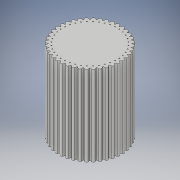
# Autodesk Inventor part: shaft
Saved by Autodesk Inventor 2019.3 (Build 233278000, 278)
## iProperties
Created: 2018-12-19
Part Number: shaft
Material: Generic
Document SubType Name: Modeling
Designer: Frienddo
Density: 1 g/cm^3
Appearance: Default
Author: Frienddo
Autodesk Inventor part; units mm, degrees
ref_plane "YZ Plane" through (0, 0, 0) normal (1, 0, 0) x (0, 1, 0)
ref_plane "XZ Plane" through (0, 0, 0) normal (0, 1, 0) x (-1, 0, 0)
ref_plane "XY Plane" through (0, 0, 0) normal (0, 0, 1) x (1, 0, 0)
sketch "Sketch1" plane through (0, 0, 0) normal (0, 1, 0) x (-1, 0, 0)
  line L0 (2.2915, -4.4974) -> (1.9316, -4.6633)
  line L1 (1.9316, -4.6633) -> (1.5598, -4.8005)
  line L2 (1.5598, -4.8005) -> (1.1783, -4.9081)
  line L3 (1.1783, -4.9081) -> (0.7896, -4.9854)
  line L4 (0.7896, -4.9854) -> (0.396, -5.032)
  line L5 (0.396, -5.032) -> (0, -5.0475)
  line L6 (0, -5.0475) -> (-0.396, -5.032)
  line L7 (-0.396, -5.032) -> (-0.7896, -4.9854)
  line L8 (-0.7896, -4.9854) -> (-1.1783, -4.9081)
  line L9 (-1.1783, -4.9081) -> (-1.5598, -4.8005)
  line L10 (-1.5598, -4.8005) -> (-1.9316, -4.6633)
  line L11 (-1.9316, -4.6633) -> (-2.2915, -4.4974)
  line L12 (-2.2915, -4.4974) -> (-2.6373, -4.3037)
  line L13 (-2.6373, -4.3037) -> (-2.9669, -4.0835)
  line L14 (-2.9669, -4.0835) -> (-3.2781, -3.8382)
  line L15 (-3.2781, -3.8382) -> (-3.5692, -3.5692)
  line L16 (-3.5692, -3.5692) -> (-3.8382, -3.2781)
  line L17 (-3.8382, -3.2781) -> (-4.0835, -2.9669)
  line L18 (-4.0835, -2.9669) -> (-4.3037, -2.6373)
  line L19 (-4.3037, -2.6373) -> (-4.4974, -2.2915)
  line L20 (-4.4974, -2.2915) -> (-4.6633, -1.9316)
  line L21 (-4.6633, -1.9316) -> (-4.8005, -1.5598)
  line L22 (-4.8005, -1.5598) -> (-4.9081, -1.1783)
  line L23 (-4.9081, -1.1783) -> (-4.9854, -0.7896)
  line L24 (-4.9854, -0.7896) -> (-5.032, -0.396)
  line L25 (-5.032, -0.396) -> (-5.0475, 0)
  line L26 (-5.0475, 0) -> (-5.032, 0.396)
  line L27 (-5.032, 0.396) -> (-4.9854, 0.7896)
  line L28 (-4.9854, 0.7896) -> (-4.9081, 1.1783)
  line L29 (-4.9081, 1.1783) -> (-4.8005, 1.5598)
  line L30 (-4.8005, 1.5598) -> (-4.6633, 1.9316)
  line L31 (-4.6633, 1.9316) -> (-4.4974, 2.2915)
  line L32 (-4.4974, 2.2915) -> (-4.3037, 2.6373)
  line L33 (-4.3037, 2.6373) -> (-4.0835, 2.9669)
  line L34 (-4.0835, 2.9669) -> (-3.8382, 3.2781)
  line L35 (-3.8382, 3.2781) -> (-3.5692, 3.5692)
  line L36 (-3.5692, 3.5692) -> (-3.2781, 3.8382)
  line L37 (-3.2781, 3.8382) -> (-2.9669, 4.0835)
  line L38 (-2.9669, 4.0835) -> (-2.6373, 4.3037)
  line L39 (-2.6373, 4.3037) -> (-2.2915, 4.4974)
  line L40 (-2.2915, 4.4974) -> (-1.9316, 4.6633)
  line L41 (-1.9316, 4.6633) -> (-1.5598, 4.8005)
  line L42 (-1.5598, 4.8005) -> (-1.1783, 4.9081)
  line L43 (-1.1783, 4.9081) -> (-0.7896, 4.9854)
  line L44 (-0.7896, 4.9854) -> (-0.396, 5.032)
  line L45 (-0.396, 5.032) -> (0, 5.0475)
  line L46 (0, 5.0475) -> (0.396, 5.032)
  line L47 (0.396, 5.032) -> (0.7896, 4.9854)
  line L48 (0.7896, 4.9854) -> (1.1783, 4.9081)
  line L49 (1.1783, 4.9081) -> (1.5598, 4.8005)
  line L50 (1.5598, 4.8005) -> (1.9316, 4.6633)
  line L51 (1.9316, 4.6633) -> (2.2915, 4.4974)
  line L52 (2.2915, 4.4974) -> (2.6373, 4.3037)
  line L53 (2.6373, 4.3037) -> (2.9669, 4.0835)
  line L54 (2.9669, 4.0835) -> (3.2781, 3.8382)
  line L55 (3.2781, 3.8382) -> (3.5692, 3.5692)
  line L56 (3.5692, 3.5692) -> (3.8382, 3.2781)
  line L57 (3.8382, 3.2781) -> (4.0835, 2.9669)
  line L58 (4.0835, 2.9669) -> (4.3037, 2.6373)
  line L59 (4.3037, 2.6373) -> (4.4974, 2.2915)
  line L60 (4.4974, 2.2915) -> (4.6633, 1.9316)
  line L61 (4.6633, 1.9316) -> (4.8005, 1.5598)
  line L62 (4.8005, 1.5598) -> (4.9081, 1.1783)
  line L63 (4.9081, 1.1783) -> (4.9854, 0.7896)
  line L64 (4.9854, 0.7896) -> (5.032, 0.396)
  line L65 (5.032, 0.396) -> (5.0475, 0)
  line L66 (5.0475, 0) -> (5.032, -0.396)
  line L67 (5.032, -0.396) -> (4.9854, -0.7896)
  line L68 (4.9854, -0.7896) -> (4.9081, -1.1783)
  line L69 (4.9081, -1.1783) -> (4.8005, -1.5598)
  line L70 (4.8005, -1.5598) -> (4.6633, -1.9316)
  line L71 (4.6633, -1.9316) -> (4.4974, -2.2915)
  line L72 (4.4974, -2.2915) -> (4.3037, -2.6373)
  line L73 (4.3037, -2.6373) -> (4.0835, -2.9669)
  line L74 (4.0835, -2.9669) -> (3.8382, -3.2781)
  line L75 (3.8382, -3.2781) -> (3.5692, -3.5692)
  line L76 (3.5692, -3.5692) -> (3.2781, -3.8382)
  line L77 (3.2781, -3.8382) -> (2.9669, -4.0835)
  line L78 (2.9669, -4.0835) -> (2.6373, -4.3037)
  line L79 (2.6373, -4.3037) -> (2.2915, -4.4974)
  line L80 (0, 0) -> (0, -5.0475) construction
  circle A0 centre (0, -5.0475) radius 0.25
  circle A1 centre (-0.7896, -4.9854) radius 0.25
  circle A2 centre (-0.4486, -5.7003) radius 0.25
  line L81 (0, -5.0475) -> (-0.4486, -5.7003) construction
  line L82 (-0.4486, -5.7003) -> (-0.7896, -4.9854) construction
  line L83 (-0.4486, -5.7003) -> (0, 0) construction
  line L84 (0.206, -5.1891) -> (-0.2426, -5.8419)
  line L85 (-0.206, -4.9059) -> (-0.6547, -5.5587)
  line L86 (-0.223, -5.5927) -> (-0.564, -4.8778)
  line L87 (-0.6743, -5.8079) -> (-1.0153, -5.093)
  line L88 (0, 0) -> (0.4486, -5.7003) construction
  circle A3 centre (0.4486, -5.7003) radius 0.25
  line L89 (-0.206, -5.1891) -> (0, -5.4889)
  line L90 (0.6547, -5.5587) -> (0.206, -4.9059)
  line L91 (0, -5.0475) -> (0.4486, -5.7003) construction
  line L92 (0, -5.4889) -> (0.2426, -5.8419)
  circle A4 centre (0, 0) radius 3.4236 construction
  circle A5 centre (0, 0) radius 3.4236 construction
  circle A6 centre (1.3348, -5.5599) radius 0.25
  line L93 (0.8587, -5.4213) -> (1.1535, -5.732)
  line L94 (1.5162, -5.3878) -> (0.971, -4.8133)
  line L95 (1.0153, -5.093) -> (0.6743, -5.8079)
  line L96 (0.6083, -5.1575) -> (0.8587, -5.4213)
  circle A7 centre (0.7896, -4.9854) radius 0.25
  line L97 (0.564, -4.8778) -> (0.223, -5.5927)
  circle A8 centre (0.4486, -5.7003) radius 0.25
  circle A9 centre (0, 0) radius 3.4236 construction
  circle A10 centre (2.1882, -5.2827) radius 0.25
  line L98 (1.6962, -5.2203) -> (2.036, -5.481)
  line L99 (2.3403, -5.0843) -> (1.712, -4.6022)
  line L100 (1.7995, -4.8715) -> (1.5745, -5.6309)
  line L101 (1.4076, -4.9988) -> (1.6962, -5.2203)
  circle A11 centre (1.5598, -4.8005) radius 0.25
  line L102 (1.3201, -4.7295) -> (1.0951, -5.4889)
  circle A12 centre (1.3348, -5.5599) radius 0.25
  circle A13 centre (0, 0) radius 3.4236 construction
  circle A14 centre (2.9876, -4.8753) radius 0.25
  line L103 (2.4919, -4.8907) -> (2.8683, -5.095)
  line L104 (3.1069, -4.6556) -> (2.4108, -4.2777)
  line L105 (2.5394, -4.53) -> (2.436, -5.3153)
  line L106 (2.1722, -4.7171) -> (2.4919, -4.8907)
  circle A15 centre (2.2915, -4.4974) radius 0.25
  line L107 (2.0437, -4.4648) -> (1.9403, -5.25)
  circle A16 centre (2.1882, -5.2827) radius 0.25
  circle A17 centre (0, 0) radius 3.4236 construction
  circle A18 centre (3.7135, -4.3479) radius 0.25
  line L108 (3.2263, -4.4406) -> (3.63, -4.5836)
  line L109 (3.7969, -4.1123) -> (3.0503, -3.8479)
  line L110 (3.2168, -4.077) -> (3.2375, -4.8688)
  line L111 (2.8834, -4.3192) -> (3.2263, -4.4406)
  circle A19 centre (2.9669, -4.0835) radius 0.25
  line L112 (2.717, -4.0901) -> (2.7377, -4.8819)
  circle A20 centre (2.9876, -4.8753) radius 0.25
  circle A21 centre (0, 0) radius 3.4236 construction
  circle A22 centre (4.3479, -3.7135) radius 0.25
  line L113 (3.8813, -3.8813) -> (4.3024, -3.9593)
  line L114 (4.3935, -3.4677) -> (3.6147, -3.3233)
  line L115 (3.815, -3.5236) -> (3.9593, -4.3024)
  line L116 (3.5236, -3.815) -> (3.8813, -3.8813)
  circle A23 centre (3.5692, -3.5692) radius 0.25
  line L117 (3.3233, -3.6147) -> (3.4677, -4.3935)
  circle A24 centre (3.7135, -4.3479) radius 0.25
  circle A25 centre (0, 0) radius 3.4236 construction
  circle A26 centre (4.8753, -2.9876) radius 0.25
  line L118 (4.4406, -3.2263) -> (4.8688, -3.2375)
  line L119 (4.8819, -2.7377) -> (4.0901, -2.717)
  line L120 (4.3192, -2.8834) -> (4.5836, -3.63)
  line L121 (4.077, -3.2168) -> (4.4406, -3.2263)
  circle A27 centre (4.0835, -2.9669) radius 0.25
  line L122 (3.8479, -3.0503) -> (4.1123, -3.7969)
  circle A28 centre (4.3479, -3.7135) radius 0.25
  circle A29 centre (0, 0) radius 3.4236 construction
  circle A30 centre (5.2827, -2.1882) radius 0.25
  line L123 (4.8907, -2.4919) -> (5.3153, -2.436)
  line L124 (5.25, -1.9403) -> (4.4648, -2.0437)
  line L125 (4.7171, -2.1722) -> (5.095, -2.8683)
  line L126 (4.53, -2.5394) -> (4.8907, -2.4919)
  circle A31 centre (4.4974, -2.2915) radius 0.25
  line L127 (4.2777, -2.4108) -> (4.6556, -3.1069)
  circle A32 centre (4.8753, -2.9876) radius 0.25
  circle A33 centre (0, 0) radius 3.4236 construction
  circle A34 centre (5.5599, -1.3348) radius 0.25
  line L128 (5.2203, -1.6962) -> (5.6309, -1.5745)
  line L129 (5.4889, -1.0951) -> (4.7295, -1.3201)
  line L130 (4.9988, -1.4076) -> (5.481, -2.036)
  line L131 (4.8715, -1.7995) -> (5.2203, -1.6962)
  circle A35 centre (4.8005, -1.5598) radius 0.25
  line L132 (4.6022, -1.712) -> (5.0843, -2.3403)
  circle A36 centre (5.2827, -2.1882) radius 0.25
  circle A37 centre (0, 0) radius 3.4236 construction
  circle A38 centre (5.7003, -0.4486) radius 0.25
  line L133 (5.4213, -0.8587) -> (5.8079, -0.6743)
  line L134 (5.5927, -0.223) -> (4.8778, -0.564)
  line L135 (5.1575, -0.6083) -> (5.732, -1.1535)
  line L136 (5.093, -1.0153) -> (5.4213, -0.8587)
  circle A39 centre (4.9854, -0.7896) radius 0.25
  line L137 (4.8133, -0.971) -> (5.3878, -1.5162)
  circle A40 centre (5.5599, -1.3348) radius 0.25
  circle A41 centre (0, 0) radius 3.4236 construction
  circle A42 centre (5.7003, 0.4486) radius 0.25
  line L138 (5.4889, 0) -> (5.8419, 0.2426)
  line L139 (5.5587, 0.6547) -> (4.9059, 0.206)
  line L140 (5.1891, 0.206) -> (5.8419, -0.2426)
  line L141 (5.1891, -0.206) -> (5.4889, 0)
  circle A43 centre (5.0475, 0) radius 0.25
  line L142 (4.9059, -0.206) -> (5.5587, -0.6547)
  circle A44 centre (5.7003, -0.4486) radius 0.25
  circle A45 centre (0, 0) radius 3.4236 construction
  circle A46 centre (5.5599, 1.3348) radius 0.25
  line L143 (5.4213, 0.8587) -> (5.732, 1.1535)
  line L144 (5.3878, 1.5162) -> (4.8133, 0.971)
  line L145 (5.093, 1.0153) -> (5.8079, 0.6743)
  line L146 (5.1575, 0.6083) -> (5.4213, 0.8587)
  circle A47 centre (4.9854, 0.7896) radius 0.25
  line L147 (4.8778, 0.564) -> (5.5927, 0.223)
  circle A48 centre (5.7003, 0.4486) radius 0.25
  circle A49 centre (0, 0) radius 3.4236 construction
  circle A50 centre (5.2827, 2.1882) radius 0.25
  line L148 (5.2203, 1.6962) -> (5.481, 2.036)
  line L149 (5.0843, 2.3403) -> (4.6022, 1.712)
  line L150 (4.8715, 1.7995) -> (5.6309, 1.5745)
  line L151 (4.9988, 1.4076) -> (5.2203, 1.6962)
  circle A51 centre (4.8005, 1.5598) radius 0.25
  line L152 (4.7295, 1.3201) -> (5.4889, 1.0951)
  circle A52 centre (5.5599, 1.3348) radius 0.25
  circle A53 centre (0, 0) radius 3.4236 construction
  circle A54 centre (4.8753, 2.9876) radius 0.25
  line L153 (4.8907, 2.4919) -> (5.095, 2.8683)
  line L154 (4.6556, 3.1069) -> (4.2777, 2.4108)
  line L155 (4.53, 2.5394) -> (5.3153, 2.436)
  line L156 (4.7171, 2.1722) -> (4.8907, 2.4919)
  circle A55 centre (4.4974, 2.2915) radius 0.25
  line L157 (4.4648, 2.0437) -> (5.25, 1.9403)
  circle A56 centre (5.2827, 2.1882) radius 0.25
  circle A57 centre (0, 0) radius 3.4236 construction
  circle A58 centre (4.3479, 3.7135) radius 0.25
  line L158 (4.4406, 3.2263) -> (4.5836, 3.63)
  line L159 (4.1123, 3.7969) -> (3.8479, 3.0503)
  line L160 (4.077, 3.2168) -> (4.8688, 3.2375)
  line L161 (4.3192, 2.8834) -> (4.4406, 3.2263)
  circle A59 centre (4.0835, 2.9669) radius 0.25
  line L162 (4.0901, 2.717) -> (4.8819, 2.7377)
  circle A60 centre (4.8753, 2.9876) radius 0.25
  circle A61 centre (0, 0) radius 3.4236 construction
  circle A62 centre (3.7135, 4.3479) radius 0.25
  line L163 (3.8813, 3.8813) -> (3.9593, 4.3024)
  line L164 (3.4677, 4.3935) -> (3.3233, 3.6147)
  line L165 (3.5236, 3.815) -> (4.3024, 3.9593)
  line L166 (3.815, 3.5236) -> (3.8813, 3.8813)
  circle A63 centre (3.5692, 3.5692) radius 0.25
  line L167 (3.6147, 3.3233) -> (4.3935, 3.4677)
  circle A64 centre (4.3479, 3.7135) radius 0.25
  circle A65 centre (0, 0) radius 3.4236 construction
  circle A66 centre (2.9876, 4.8753) radius 0.25
  line L168 (3.2263, 4.4406) -> (3.2375, 4.8688)
  line L169 (2.7377, 4.8819) -> (2.717, 4.0901)
  line L170 (2.8834, 4.3192) -> (3.63, 4.5836)
  line L171 (3.2168, 4.077) -> (3.2263, 4.4406)
  circle A67 centre (2.9669, 4.0835) radius 0.25
  line L172 (3.0503, 3.8479) -> (3.7969, 4.1123)
  circle A68 centre (3.7135, 4.3479) radius 0.25
  circle A69 centre (0, 0) radius 3.4236 construction
  circle A70 centre (2.1882, 5.2827) radius 0.25
  line L173 (2.4919, 4.8907) -> (2.436, 5.3153)
  line L174 (1.9403, 5.25) -> (2.0437, 4.4648)
  line L175 (2.1722, 4.7171) -> (2.8683, 5.095)
  line L176 (2.5394, 4.53) -> (2.4919, 4.8907)
  circle A71 centre (2.2915, 4.4974) radius 0.25
  line L177 (2.4108, 4.2777) -> (3.1069, 4.6556)
  circle A72 centre (2.9876, 4.8753) radius 0.25
  circle A73 centre (0, 0) radius 3.4236 construction
  circle A74 centre (1.3348, 5.5599) radius 0.25
  line L178 (1.6962, 5.2203) -> (1.5745, 5.6309)
  line L179 (1.0951, 5.4889) -> (1.3201, 4.7295)
  line L180 (1.4076, 4.9988) -> (2.036, 5.481)
  line L181 (1.7995, 4.8715) -> (1.6962, 5.2203)
  circle A75 centre (1.5598, 4.8005) radius 0.25
  line L182 (1.712, 4.6022) -> (2.3403, 5.0843)
  circle A76 centre (2.1882, 5.2827) radius 0.25
  circle A77 centre (0, 0) radius 3.4236 construction
  circle A78 centre (0.4486, 5.7003) radius 0.25
  line L183 (0.8587, 5.4213) -> (0.6743, 5.8079)
  line L184 (0.223, 5.5927) -> (0.564, 4.8778)
  line L185 (0.6083, 5.1575) -> (1.1535, 5.732)
  line L186 (1.0153, 5.093) -> (0.8587, 5.4213)
  circle A79 centre (0.7896, 4.9854) radius 0.25
  line L187 (0.971, 4.8133) -> (1.5162, 5.3878)
  circle A80 centre (1.3348, 5.5599) radius 0.25
  circle A81 centre (0, 0) radius 3.4236 construction
  circle A82 centre (-0.4486, 5.7003) radius 0.25
  line L188 (0, 5.4889) -> (-0.2426, 5.8419)
  line L189 (-0.6547, 5.5587) -> (-0.206, 4.9059)
  line L190 (-0.206, 5.1891) -> (0.2426, 5.8419)
  line L191 (0.206, 5.1891) -> (0, 5.4889)
  circle A83 centre (0, 5.0475) radius 0.25
  line L192 (0.206, 4.9059) -> (0.6547, 5.5587)
  circle A84 centre (0.4486, 5.7003) radius 0.25
  circle A85 centre (0, 0) radius 3.4236 construction
  circle A86 centre (-1.3348, 5.5599) radius 0.25
  line L193 (-0.8587, 5.4213) -> (-1.1535, 5.732)
  line L194 (-1.5162, 5.3878) -> (-0.971, 4.8133)
  line L195 (-1.0153, 5.093) -> (-0.6743, 5.8079)
  line L196 (-0.6083, 5.1575) -> (-0.8587, 5.4213)
  circle A87 centre (-0.7896, 4.9854) radius 0.25
  line L197 (-0.564, 4.8778) -> (-0.223, 5.5927)
  circle A88 centre (-0.4486, 5.7003) radius 0.25
  circle A89 centre (0, 0) radius 3.4236 construction
  circle A90 centre (-2.1882, 5.2827) radius 0.25
  line L198 (-1.6962, 5.2203) -> (-2.036, 5.481)
  line L199 (-2.3403, 5.0843) -> (-1.712, 4.6022)
  line L200 (-1.7995, 4.8715) -> (-1.5745, 5.6309)
  line L201 (-1.4076, 4.9988) -> (-1.6962, 5.2203)
  circle A91 centre (-1.5598, 4.8005) radius 0.25
  line L202 (-1.3201, 4.7295) -> (-1.0951, 5.4889)
  circle A92 centre (-1.3348, 5.5599) radius 0.25
  circle A93 centre (0, 0) radius 3.4236 construction
  circle A94 centre (-2.9876, 4.8753) radius 0.25
  line L203 (-2.4919, 4.8907) -> (-2.8683, 5.095)
  line L204 (-3.1069, 4.6556) -> (-2.4108, 4.2777)
  line L205 (-2.5394, 4.53) -> (-2.436, 5.3153)
  line L206 (-2.1722, 4.7171) -> (-2.4919, 4.8907)
  circle A95 centre (-2.2915, 4.4974) radius 0.25
  line L207 (-2.0437, 4.4648) -> (-1.9403, 5.25)
  circle A96 centre (-2.1882, 5.2827) radius 0.25
  circle A97 centre (0, 0) radius 3.4236 construction
  circle A98 centre (-3.7135, 4.3479) radius 0.25
  line L208 (-3.2263, 4.4406) -> (-3.63, 4.5836)
  line L209 (-3.7969, 4.1123) -> (-3.0503, 3.8479)
  line L210 (-3.2168, 4.077) -> (-3.2375, 4.8688)
  line L211 (-2.8834, 4.3192) -> (-3.2263, 4.4406)
  circle A99 centre (-2.9669, 4.0835) radius 0.25
  line L212 (-2.717, 4.0901) -> (-2.7377, 4.8819)
  circle A100 centre (-2.9876, 4.8753) radius 0.25
  circle A101 centre (0, 0) radius 3.4236 construction
  circle A102 centre (-4.3479, 3.7135) radius 0.25
  line L213 (-3.8813, 3.8813) -> (-4.3024, 3.9593)
  line L214 (-4.3935, 3.4677) -> (-3.6147, 3.3233)
  line L215 (-3.815, 3.5236) -> (-3.9593, 4.3024)
  line L216 (-3.5236, 3.815) -> (-3.8813, 3.8813)
  circle A103 centre (-3.5692, 3.5692) radius 0.25
  line L217 (-3.3233, 3.6147) -> (-3.4677, 4.3935)
  circle A104 centre (-3.7135, 4.3479) radius 0.25
  circle A105 centre (0, 0) radius 3.4236 construction
  circle A106 centre (-4.8753, 2.9876) radius 0.25
  line L218 (-4.4406, 3.2263) -> (-4.8688, 3.2375)
  line L219 (-4.8819, 2.7377) -> (-4.0901, 2.717)
  line L220 (-4.3192, 2.8834) -> (-4.5836, 3.63)
  line L221 (-4.077, 3.2168) -> (-4.4406, 3.2263)
  circle A107 centre (-4.0835, 2.9669) radius 0.25
  line L222 (-3.8479, 3.0503) -> (-4.1123, 3.7969)
  circle A108 centre (-4.3479, 3.7135) radius 0.25
  circle A109 centre (0, 0) radius 3.4236 construction
  circle A110 centre (-5.2827, 2.1882) radius 0.25
  line L223 (-4.8907, 2.4919) -> (-5.3153, 2.436)
  line L224 (-5.25, 1.9403) -> (-4.4648, 2.0437)
  line L225 (-4.7171, 2.1722) -> (-5.095, 2.8683)
  line L226 (-4.53, 2.5394) -> (-4.8907, 2.4919)
  circle A111 centre (-4.4974, 2.2915) radius 0.25
  line L227 (-4.2777, 2.4108) -> (-4.6556, 3.1069)
  circle A112 centre (-4.8753, 2.9876) radius 0.25
  circle A113 centre (0, 0) radius 3.4236 construction
  circle A114 centre (-5.5599, 1.3348) radius 0.25
  line L228 (-5.2203, 1.6962) -> (-5.6309, 1.5745)
  line L229 (-5.4889, 1.0951) -> (-4.7295, 1.3201)
  line L230 (-4.9988, 1.4076) -> (-5.481, 2.036)
  line L231 (-4.8715, 1.7995) -> (-5.2203, 1.6962)
  circle A115 centre (-4.8005, 1.5598) radius 0.25
  line L232 (-4.6022, 1.712) -> (-5.0843, 2.3403)
  circle A116 centre (-5.2827, 2.1882) radius 0.25
  circle A117 centre (0, 0) radius 3.4236 construction
  circle A118 centre (-5.7003, 0.4486) radius 0.25
  line L233 (-5.4213, 0.8587) -> (-5.8079, 0.6743)
  line L234 (-5.5927, 0.223) -> (-4.8778, 0.564)
  line L235 (-5.1575, 0.6083) -> (-5.732, 1.1535)
  line L236 (-5.093, 1.0153) -> (-5.4213, 0.8587)
  circle A119 centre (-4.9854, 0.7896) radius 0.25
  line L237 (-4.8133, 0.971) -> (-5.3878, 1.5162)
  circle A120 centre (-5.5599, 1.3348) radius 0.25
  circle A121 centre (0, 0) radius 3.4236 construction
  circle A122 centre (-5.7003, -0.4486) radius 0.25
  line L238 (-5.4889, 0) -> (-5.8419, -0.2426)
  line L239 (-5.5587, -0.6547) -> (-4.9059, -0.206)
  line L240 (-5.1891, -0.206) -> (-5.8419, 0.2426)
  line L241 (-5.1891, 0.206) -> (-5.4889, 0)
  circle A123 centre (-5.0475, 0) radius 0.25
  line L242 (-4.9059, 0.206) -> (-5.5587, 0.6547)
  circle A124 centre (-5.7003, 0.4486) radius 0.25
  circle A125 centre (0, 0) radius 3.4236 construction
  circle A126 centre (-5.5599, -1.3348) radius 0.25
  line L243 (-5.4213, -0.8587) -> (-5.732, -1.1535)
  line L244 (-5.3878, -1.5162) -> (-4.8133, -0.971)
  line L245 (-5.093, -1.0153) -> (-5.8079, -0.6743)
  line L246 (-5.1575, -0.6083) -> (-5.4213, -0.8587)
  circle A127 centre (-4.9854, -0.7896) radius 0.25
  line L247 (-4.8778, -0.564) -> (-5.5927, -0.223)
  circle A128 centre (-5.7003, -0.4486) radius 0.25
  circle A129 centre (0, 0) radius 3.4236 construction
  circle A130 centre (-5.2827, -2.1882) radius 0.25
  line L248 (-5.2203, -1.6962) -> (-5.481, -2.036)
  line L249 (-5.0843, -2.3403) -> (-4.6022, -1.712)
  line L250 (-4.8715, -1.7995) -> (-5.6309, -1.5745)
  line L251 (-4.9988, -1.4076) -> (-5.2203, -1.6962)
  circle A131 centre (-4.8005, -1.5598) radius 0.25
  line L252 (-4.7295, -1.3201) -> (-5.4889, -1.0951)
  circle A132 centre (-5.5599, -1.3348) radius 0.25
  circle A133 centre (0, 0) radius 3.4236 construction
  circle A134 centre (-4.8753, -2.9876) radius 0.25
  line L253 (-4.8907, -2.4919) -> (-5.095, -2.8683)
  line L254 (-4.6556, -3.1069) -> (-4.2777, -2.4108)
  line L255 (-4.53, -2.5394) -> (-5.3153, -2.436)
  line L256 (-4.7171, -2.1722) -> (-4.8907, -2.4919)
  circle A135 centre (-4.4974, -2.2915) radius 0.25
  line L257 (-4.4648, -2.0437) -> (-5.25, -1.9403)
  circle A136 centre (-5.2827, -2.1882) radius 0.25
  circle A137 centre (0, 0) radius 3.4236 construction
  circle A138 centre (-4.3479, -3.7135) radius 0.25
  line L258 (-4.4406, -3.2263) -> (-4.5836, -3.63)
  line L259 (-4.1123, -3.7969) -> (-3.8479, -3.0503)
  line L260 (-4.077, -3.2168) -> (-4.8688, -3.2375)
  line L261 (-4.3192, -2.8834) -> (-4.4406, -3.2263)
  circle A139 centre (-4.0835, -2.9669) radius 0.25
  line L262 (-4.0901, -2.717) -> (-4.8819, -2.7377)
  circle A140 centre (-4.8753, -2.9876) radius 0.25
  circle A141 centre (0, 0) radius 3.4236 construction
  circle A142 centre (-3.7135, -4.3479) radius 0.25
  line L263 (-3.8813, -3.8813) -> (-3.9593, -4.3024)
  line L264 (-3.4677, -4.3935) -> (-3.3233, -3.6147)
  line L265 (-3.5236, -3.815) -> (-4.3024, -3.9593)
  line L266 (-3.815, -3.5236) -> (-3.8813, -3.8813)
  circle A143 centre (-3.5692, -3.5692) radius 0.25
  line L267 (-3.6147, -3.3233) -> (-4.3935, -3.4677)
  circle A144 centre (-4.3479, -3.7135) radius 0.25
  circle A145 centre (0, 0) radius 3.4236 construction
  circle A146 centre (-2.9876, -4.8753) radius 0.25
  line L268 (-3.2263, -4.4406) -> (-3.2375, -4.8688)
  line L269 (-2.7377, -4.8819) -> (-2.717, -4.0901)
  line L270 (-2.8834, -4.3192) -> (-3.63, -4.5836)
  line L271 (-3.2168, -4.077) -> (-3.2263, -4.4406)
  circle A147 centre (-2.9669, -4.0835) radius 0.25
  line L272 (-3.0503, -3.8479) -> (-3.7969, -4.1123)
  circle A148 centre (-3.7135, -4.3479) radius 0.25
  circle A149 centre (0, 0) radius 3.4236 construction
  circle A150 centre (-2.1882, -5.2827) radius 0.25
  line L273 (-2.4919, -4.8907) -> (-2.436, -5.3153)
  line L274 (-1.9403, -5.25) -> (-2.0437, -4.4648)
  line L275 (-2.1722, -4.7171) -> (-2.8683, -5.095)
  line L276 (-2.5394, -4.53) -> (-2.4919, -4.8907)
  circle A151 centre (-2.2915, -4.4974) radius 0.25
  line L277 (-2.4108, -4.2777) -> (-3.1069, -4.6556)
  circle A152 centre (-2.9876, -4.8753) radius 0.25
  circle A153 centre (0, 0) radius 3.4236 construction
  circle A154 centre (-1.3348, -5.5599) radius 0.25
  line L278 (-1.6962, -5.2203) -> (-1.5745, -5.6309)
  line L279 (-1.0951, -5.4889) -> (-1.3201, -4.7295)
  line L280 (-1.4076, -4.9988) -> (-2.036, -5.481)
  line L281 (-1.7995, -4.8715) -> (-1.6962, -5.2203)
  circle A155 centre (-1.5598, -4.8005) radius 0.25
  line L282 (-1.712, -4.6022) -> (-2.3403, -5.0843)
  circle A156 centre (-2.1882, -5.2827) radius 0.25
  circle A157 centre (0, 0) radius 3.4236 construction
  circle A158 centre (-0.4486, -5.7003) radius 0.25
  line L283 (-0.8587, -5.4213) -> (-0.6743, -5.8079)
  line L284 (-0.223, -5.5927) -> (-0.564, -4.8778)
  line L285 (-0.6083, -5.1575) -> (-1.1535, -5.732)
  line L286 (-1.0153, -5.093) -> (-0.8587, -5.4213)
  circle A159 centre (-0.7896, -4.9854) radius 0.25
  line L287 (-0.971, -4.8133) -> (-1.5162, -5.3878)
  circle A160 centre (-1.3348, -5.5599) radius 0.25
  point P0 (0.2426, -5.8419)
  point P1 (0.6547, -5.5587)
  point P2 (1.1535, -5.732)
  point P3 (1.5162, -5.3878)
  point P4 (2.036, -5.481)
  point P5 (2.3403, -5.0843)
  point P6 (2.8683, -5.095)
  point P7 (3.1069, -4.6556)
  point P8 (3.63, -4.5836)
  point P9 (3.7969, -4.1123)
  point P10 (4.3024, -3.9593)
  point P11 (4.3935, -3.4677)
  point P12 (4.8688, -3.2375)
  point P13 (4.8819, -2.7377)
  point P14 (5.3153, -2.436)
  point P15 (5.25, -1.9403)
  point P16 (5.6309, -1.5745)
  point P17 (5.4889, -1.0951)
  point P18 (5.8079, -0.6743)
  point P19 (5.5927, -0.223)
  point P20 (5.8419, 0.2426)
  point P21 (5.5587, 0.6547)
  point P22 (5.732, 1.1535)
  point P23 (5.3878, 1.5162)
  point P24 (5.481, 2.036)
  point P25 (5.0843, 2.3403)
  point P26 (5.095, 2.8683)
  point P27 (4.6556, 3.1069)
  point P28 (4.5836, 3.63)
  point P29 (4.1123, 3.7969)
  point P30 (3.9593, 4.3024)
  point P31 (3.4677, 4.3935)
  point P32 (3.2375, 4.8688)
  point P33 (2.7377, 4.8819)
  point P34 (2.436, 5.3153)
  point P35 (1.9403, 5.25)
  point P36 (1.5745, 5.6309)
  point P37 (1.0951, 5.4889)
  point P38 (0.6743, 5.8079)
  point P39 (0.223, 5.5927)
  point P40 (-0.2426, 5.8419)
  point P41 (-0.6547, 5.5587)
  point P42 (-1.1535, 5.732)
  point P43 (-1.5162, 5.3878)
  point P44 (-2.036, 5.481)
  point P45 (-2.3403, 5.0843)
  point P46 (-2.8683, 5.095)
  point P47 (-3.1069, 4.6556)
  point P48 (-3.63, 4.5836)
  point P49 (-3.7969, 4.1123)
  point P50 (-4.3024, 3.9593)
  point P51 (-4.3935, 3.4677)
  point P52 (-4.8688, 3.2375)
  point P53 (-4.8819, 2.7377)
  point P54 (-5.3153, 2.436)
  point P55 (-5.25, 1.9403)
  point P56 (-5.6309, 1.5745)
  point P57 (-5.4889, 1.0951)
  point P58 (-5.8079, 0.6743)
  point P59 (-5.5927, 0.223)
  point P60 (-5.8419, -0.2426)
  point P61 (-5.5587, -0.6547)
  point P62 (-5.732, -1.1535)
  point P63 (-5.3878, -1.5162)
  point P64 (-5.481, -2.036)
  point P65 (-5.0843, -2.3403)
  point P66 (-5.095, -2.8683)
  point P67 (-4.6556, -3.1069)
  point P68 (-4.5836, -3.63)
  point P69 (-4.1123, -3.7969)
  point P70 (-3.9593, -4.3024)
  point P71 (-3.4677, -4.3935)
  point P72 (-3.2375, -4.8688)
  point P73 (-2.7377, -4.8819)
  point P74 (-2.436, -5.3153)
  point P75 (-1.9403, -5.25)
  point P76 (-1.5745, -5.6309)
  point P77 (-1.0951, -5.4889)
  dimension "d3" = 5.0475
  dimension "d4" = 0.5
  dimension "d5" = 0.5
  dimension "d6" = 0.5
  dimension "d7" = 60
  dimension "d8" = 0.5
  dimension "d9" = 30
  dimension "d12" = 360
  constraints: 576 end point, 402 point on circle, 161 centre point, 42 point on line, 14 tangent, 7 coincident, 1 vertical, 1120 other
  measures "d3" distance of L80.start L5.end
  measures "d4" diameter of A0
  measures "d5" diameter of A1
  measures "d6" diameter of A2
  measures "d7" angle of L82 L81
  measures "d8" diameter of A3
  measures "d9" angle of L88 L91
extrude "Extrusion2" add sketch "Sketch1" along normal blind 15 contours L79 A15 L0 | L0 A15 L79 | A15 L106 L105 A10 L99 L107 L0 | L0 L107 A15 | A15 L104 L79 | L79 L104 L112 A14 L103 L105 A15 | L0 L1 L99 A11 L102 L2 L3 L94 A7 L97 L4 L5 L90 A0 L85 L6 L7 L86 A1 L287 L8 L9 L279 A155 L282 L10 L11 L274 A151 L277 L12 L13 L269 A147 L272 L14 L15 L264 A143 L267 L16 L17 L259 A139 L262 L18 L19 L254 A135 L257 L20 L21 L249 A131 L252 L22 L23 L244 A127 L247 L24 L25 L239 A123 L242 L26 L27 L234 A119 L237 L28 L29 L229 A115 L232 L30 L31 L224 A111 L227 L32 L33 L219 A107 L222 L34 L35 L214 A103 L217 L36 L37 L209 A99 L212 L38 L39 L204 A95 L207 L40 L41 L199 A91 L202 L42 L43 L194 A87 L197 L44 L45 L189 A83 L192 L46 L47 L184 A79 L187 L48 L49 L179 A75 L182 L50 L51 L174 A71 L177 L52 L53 L169 A67 L172 L54 L55 L164 A63 L167 L56 L57 L159 A59 L162 L58 L59 L154 A55 L157 L60 L61 L149 A51 L152 L62 L63 L144 A47 L147 L64 L65 L139 A43 L142 L66 L67 L134 A39 L137 L68 L69 L129 A35 L132 L70 L71 L124 A31 L127 L72 L73 L119 A27 L122 L74 L75 L114 A23 L117 L76 L77 L109 A19 L112 L78 L79 L104 A15 L107 | A15 L105 L106 | L107 A10 L98 L100 A11 L1 L99 | L99 A10 L107 | L112 L78 A19 L111 L110 A14 L104 | L104 A14 L112 | L1 A11 L99 | A10 | A14 | L112 A19 L78 | A11 L2 L1 | L1 L2 A11 | A19 L77 L78 | L78 L77 A19 L110 | A11 L2 L102 | L101 A11 L100 | L100 A6 L94 L102 L2 A11 L101 | A19 L110 L111 | L109 L77 A19 | L110 A19 L77 L109 L117 A18 L108 | A6 | A18 | L102 A6 L93 L95 A7 L3 L94 | L94 A6 L102 | L117 L76 A23 L116 L115 A18 L109 | L109 A18 L117 | L3 A7 L94 | L96 A7 L95 | L95 A3 L90 L97 L4 A7 L96 | L117 A23 L76 | A7 L4 L3 | L3 L4 A7 | A3 | A23 L75 L76 | L76 L75 A23 | L115 A23 L75 L114 L122 A22 L113 | L116 A23 L115 | A7 L4 L97 | L92 L84 A0 L5 L90 L97 A3 | L114 L75 A23 | A22 | L97 L90 A3 | L89 A0 L84 | L84 A2 L86 L85 L6 A0 L89 | L122 L114 A22 | A0 L6 L5 | A2 | L122 L74 A27 L121 L120 A22 L114 | L5 A0 L90 | L87 L285 A1 L7 L86 L85 A2 | A0 L5 L6 | L6 L85 A0 | L122 A27 L74 | L120 A27 L73 L119 L127 A26 L118 | L121 A27 L120 | L85 L86 A2 | L285 A154 L279 L287 L8 A1 L87 | L87 A1 L285 | A27 L73 L74 | L74 L73 A27 | A26 | A1 L8 L7 | A154 | L119 L73 A27 | L127 L119 A26 | L7 A1 L86 | A1 L7 L8 | L8 L287 A1 | L278 L280 A155 L9 L279 L287 A154 | L119 L127 L72 A31 L126 L125 A26 | L287 L279 A154 | L281 A155 L280 | L280 A150 L274 L282 L10 A155 L281 | L127 A31 L72 | L125 A31 L71 L124 L132 A30 L123 | L126 A31 L125 | A155 L10 L9 | A150 | A31 L71 L72 | L72 L71 A31 | A30 | L9 A155 L279 | L9 L10 A155 | L273 L275 A151 L11 L274 L282 A150 | L10 L282 A155 | L124 L71 A31 | L132 L124 A30 | L282 L274 A150 | L276 A151 L275 | L275 A146 L269 L277 L12 A151 L276 | L124 L132 L70 A35 L131 L130 A30 | A151 L12 L11 | A146 | L132 A35 L70 | L130 A35 L69 L129 L137 A34 L128 | L131 A35 L130 | L11 A151 L274 | L11 L12 A151 | L268 L270 A147 L13 L269 L277 A146 | L12 L277 A151 | A35 L69 L70 | L70 L69 A35 | A34 | L277 L269 A146 | L271 A147 L270 | L270 A142 L264 L272 L14 A147 L271 | L129 L69 A35 | L137 L129 A34 | A147 L14 L13 | A142 | L129 L137 L68 A39 L136 L135 A34 | L13 A147 L269 | L13 L14 A147 | L263 L265 A143 L15 L264 L272 A142 | A142 L272 L264 | L14 L272 A147 | L137 A39 L68 | L135 A39 L67 L134 L142 A38 L133 | L136 A39 L135 | L266 A143 L265 | L265 A138 L259 L267 L16 A143 L266 | A39 L67 L68 | L68 L67 A39 | A38 | A143 L16 L15 | A138 | L15 A143 L264 | L134 L67 A39 | L142 L134 A38 | L15 L16 A143 | L258 L260 A139 L17 L259 L267 A138 | A138 L267 L259 | L16 L267 A143 | L134 L142 L66 A43 L141 L140 A38 | L261 A139 L260 | L260 A134 L254 L262 L18 A139 L261 | L142 A43 L66 | L140 A43 L65 L139 L147 A42 L138 | L141 A43 L140 | A139 L18 L17 | A134 | L17 A139 L259 | A43 L65 L66 | L66 L65 A43 | A42 | L17 L18 A139 | L253 L255 A135 L19 L254 L262 A134 | A134 L262 L254 | L18 L262 A139 | L139 L65 A43 | L147 L139 A42 | L256 A135 L255 | L255 A130 L249 L257 L20 A135 L256 | L139 L147 L64 A47 L146 L145 A42 | A135 L20 L19 | A130 | L19 A135 L254 | L147 A47 L64 | L145 A47 L63 L144 L152 A46 L143 | L146 A47 L145 | L19 L20 A135 | L248 L250 A131 L21 L249 L257 A130 | A130 L257 L249 | L20 L257 A135 | A47 L63 L64 | L64 L63 A47 | A46 | L251 A131 L250 | L250 A126 L244 L252 L22 A131 L251 | L144 L63 A47 | L152 L144 A46 | A131 L22 L21 | A126 | L21 A131 L249 | L144 L152 L62 A51 L151 L150 A46 | L21 L22 A131 | L243 L245 A127 L23 L244 L252 A126 | A126 L252 L244 | L22 L252 A131 | L152 A51 L62 | L150 A51 L61 L149 L157 A50 L148 | L151 A51 L150 | L246 A127 L245 | L245 A122 L239 L247 L24 A127 L246 | A51 L61 L62 | L62 L61 A51 | A50 | A127 L24 L23 | A122 | L23 A127 L244 | L149 L61 A51 | L157 L149 A50 | L23 L24 A127 | L238 L240 A123 L25 L239 L247 A122 | A122 L247 L239 | L24 L247 A127 | L149 L157 L60 A55 L156 L155 A50 | L241 A123 L240 | L240 A118 L234 L242 L26 A123 L241 | L157 A55 L60 | L155 A55 L59 L154 L162 A54 L153 | L156 A55 L155 | A123 L26 L25 | A118 | L25 A123 L239 | A55 L59 L60 | L60 L59 A55 | A54 | L25 L26 A123 | L233 L235 A119 L27 L234 L242 A118 | A118 L242 L234 | L26 L242 A123 | L154 L59 A55 | L162 L154 A54 | L236 A119 L235 | L235 A114 L229 L237 L28 A119 L236 | L154 L162 L58 A59 L161 L160 A54 | A119 L28 L27 | A114 | L27 A119 L234 | L162 A59 L58 | L160 A59 L57 L159 L167 A58 L158 | L161 A59 L160 | L27 L28 A119 | L228 L230 A115 L29 L229 L237 A114 | A114 L237 L229 | L28 L237 A119 | A59 L57 L58 | L58 L57 A59 | A58 | L231 A115 L230 | L230 A110 L224 L232 L30 A115 L231 | L159 L57 A59 | L167 L159 A58 | A115 L30 L29 | A110 | L29 A115 L229 | L159 L167 L56 A63 L166 L165 A58 | L29 L30 A115 | L223 L225 A111 L31 L224 L232 A110 | A110 L232 L224 | L30 L232 A115 | L167 A63 L56 | L165 A63 L55 L164 L172 A62 L163 | L166 A63 L165 | L226 A111 L225 | L225 A106 L219 L227 L32 A111 L226 | A63 L55 L56 | L56 L55 A63 | A62 | A111 L32 L31 | A106 | L31 A111 L224 | L164 L55 A63 | L172 L164 A62 | L31 L32 A111 | L218 L220 A107 L33 L219 L227 A106 | A106 L227 L219 | L32 L227 A111 | L164 L172 L54 A67 L171 L170 A62 | L221 A107 L220 | L220 A102 L214 L222 L34 A107 L221 | L172 A67 L54 | L170 A67 L53 L169 L177 A66 L168 | L171 A67 L170 | A107 L34 L33 | A102 | L33 A107 L219 | A67 L53 L54 | L54 L53 A67 L171 | A66 | L33 L34 A107 | L213 L215 A103 L35 L214 L222 A102 | A102 L222 L214 | L34 L222 A107 | L169 L53 A67 | L177 L169 A66 | L216 A103 L215 | L215 A98 L209 L217 L36 A103 L216 | L169 L177 L52 A71 L176 L175 A66 | A103 L36 L35 | A98 | L35 A103 L214 | L177 A71 L52 | L175 A71 L51 L174 L182 A70 L173 | L176 A71 L175 | L35 L36 A103 | L208 L210 A99 L37 L209 L217 A98 | A98 L217 L209 | L36 L217 A103 | A71 L51 L52 | L52 L51 A71 | A70 | L211 A99 L210 | L210 A94 L204 L212 L38 A99 L211 | L174 L51 A71 | A70 L174 L182 L50 A75 L181 L180 | A99 L38 L37 | A94 | L37 A99 L209 | L182 L174 A70 | L180 A75 L49 L179 L187 A74 L178 | L181 A75 L180 | L37 L38 A99 | L203 L205 A95 L39 L204 L212 A94 | A94 L212 L204 | L38 L212 A99 | A74 | A75 L50 L49 | L206 A95 L205 | L205 A90 L199 L207 L40 A95 L206 | L182 A75 L50 | A74 L179 L187 L48 A79 L186 L185 | A75 L179 L49 | L49 L50 A75 | A95 L40 L39 | A90 | L39 A95 L204 | L187 L179 A74 | L185 A79 L47 L184 L192 A78 L183 | L186 A79 L185 | L39 L40 A95 | L198 L200 A91 L41 L199 L207 A90 | A90 L207 L199 | L40 L207 A95 | A78 | A79 L48 L47 | L201 A91 L200 | L200 A86 L194 L202 L42 A91 L201 | L187 A79 L48 | A78 L184 L192 L46 A83 L191 L190 | A79 L184 L47 | L47 L48 A79 | A91 L42 L41 | A86 | L41 A91 L199 | L192 L184 A78 | L190 A83 L45 L189 L197 A82 L188 | L191 A83 L190 | L41 L42 A91 | L193 L195 A87 L43 L194 L202 A86 | A86 L202 L194 | L42 L202 A91 | A82 | A83 L46 L45 | L196 A87 L195 | L195 A82 L189 L197 L44 A87 L196 | L192 A83 L46 | A83 L189 L45 | L45 L46 A83 | A87 L44 L43 | L43 A87 L194 | L197 L189 A82 | L43 L44 A87 | L44 L197 A87
equation "\"try\" = 2.236068"
body "Solid2"
